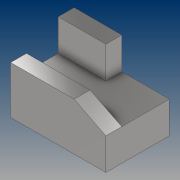
# Autodesk Inventor part: 42
Saved by Autodesk Inventor 2020.2 (Build 242310000, 310)
## iProperties
Created: 2020-09-17
Part Number: 42
Material: 鋼、碳鋼
Document SubType Name: Modeling
Designer: user
Density: 7.85 g/cm^3
Appearance: 半拋光
Mass: 463.15 g
Surface Area: 115.236 cm^2
Volume: 59 cm^3
Author: user
Autodesk Inventor part; units mm, degrees
ref_plane "YZ Plane" through (0, 0, 0) normal (1, 0, 0) x (0, 1, 0)
ref_plane "XZ Plane" through (0, 0, 0) normal (0, 1, 0) x (-1, 0, 0)
ref_plane "XY Plane" through (0, 0, 0) normal (0, 0, 1) x (1, 0, 0)
sketch "草圖1" plane through (0, 0, 0) normal (0, 1, 0) x (-1, 0, 0)
  line L0 (0, 0) -> (-60, 0)
  line L1 (-60, 0) -> (-60, 40)
  line L2 (-60, 40) -> (0, 40)
  line L3 (0, 40) -> (0, 0)
  dimension "d0" = 40
  dimension "d1" = 60
  constraints: 8 end point, 2 parallel, 1 horizontal, 1 perpendicular
  measures "d0" distance of L2.end L0.start
  measures "d1" distance of L1.end L2.end
extrude "擠出1" add sketch "草圖1" along normal blind 40
sketch "草圖2" plane through (60, 0, 40) normal (1, 0, 0) x (0, 0, -1)
  line L0 (0, 0) -> (0, 40) projected
  line L1 (0, 40) -> (40, 40) projected
  line L2 (40, 40) -> (40, 0) projected
  line L3 (40, 0) -> (0, 0) projected
  line L4 (0, 0) -> (0, 40) projected
  line L5 (0, 40) -> (40, 40) projected
  line L6 (40, 40) -> (40, 0) projected
  line L7 (40, 0) -> (0, 0) projected
  line L8 (10, 40) -> (30, 40)
  line L9 (30, 40) -> (30, 20)
  line L10 (30, 20) -> (10, 20)
  line L11 (10, 20) -> (10, 40)
  point P0 (20, 40)
  point P1 (30, 40)
  point P2 (10, 40)
  dimension "d4" = 20
  dimension "d5" = 20
  constraints: 8 end point, 2 midpoint, 2 parallel, 1 horizontal, 1 perpendicular
  measures "d4" distance of L9.end L10.end
  measures "d5" distance of L10.end L8.start
extrude "擠出2" cut sketch "草圖2" against normal through all contours L1 L9 L10 L11
sketch "草圖3" plane through (0, 0, 40) normal (0, 0, 1) x (1, 0, 0)
  line L0 (60, 40) -> (60, 0) projected
  line L1 (60, 0) -> (0, 0) projected
  line L2 (0, 0) -> (0, 40) projected
  line L3 (0, 40) -> (60, 40) projected
  line L4 (0, 20) -> (0, 40) projected
  line L5 (0, 30) -> (40, 30)
  line L6 (40, 30) -> (60, 20)
  dimension "d8" = 10
  dimension "d9" = 20
  dimension "d10" = 10
  constraints: 4 end point, 2 midpoint, 1 horizontal
  measures "d8" distance between parallel lines of L5 L3
  measures "d9" horizontal distance of L5.end L6.end
  measures "d10" vertical distance of L5.end L6.end
extrude "擠出3" cut sketch "草圖3" against normal blind 13.25 contours L0 L6 L5 L2 L3
sketch "草圖4" plane through (60, 20, 10) normal (0, 0, 1) x (1, 0, 0)
  line L0 (-60, -20) -> (-60, 0) projected
  line L1 (-60, 0) -> (-60, 20) projected
  line L2 (-60, 20) -> (0, 20) projected
  line L3 (0, 20) -> (0, 0) projected
  line L4 (0, 0) -> (0, -20) projected
  line L5 (0, -20) -> (-60, -20) projected
  line L6 (-60, 0) -> (0, 0) projected
  line L7 (-60, -20) -> (-60, 0) projected
  line L8 (-60, 0) -> (-60, 20) projected
  line L9 (-60, 20) -> (0, 20) projected
  line L10 (0, 20) -> (0, 0) projected
  line L11 (0, 0) -> (0, -20) projected
  line L12 (0, -20) -> (-60, -20) projected
  line L13 (-60, 0) -> (0, 0) projected
  line L14 (-30, 0) -> (10.073, 0)
  line L15 (10.073, 0) -> (10.073, 29.5381)
  line L16 (10.073, 29.5381) -> (-30, 29.5381)
  line L17 (-30, 29.5381) -> (-30, 0)
  point P0 (-30, 0)
  dimension "d13" = 30
  constraints: 8 end point, 2 parallel, 1 horizontal, 1 midpoint, 1 perpendicular
  measures "d13" distance between parallel lines of L17 L3
extrude "擠出4" cut sketch "草圖4" against normal blind 10 contours L17 L2 L3 L6 | L3 L2 L17 L16 L15 L14
